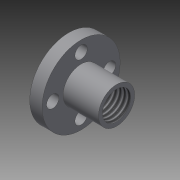
# Autodesk Inventor part: stage
Saved by Autodesk Inventor 2015 SP1 (Build 190203100, 203)
## iProperties
Created: 2016-07-08
Part Number: stage
Material: Generic
Document SubType Name: Modeling
Designer: lustinga
Density: 1 g/cm^3
Appearance: Default
Mass: 1.38148 g
Surface Area: 17.2411 cm^2
Volume: 1.38148 cm^3
Author: lustinga
Autodesk Inventor part; units mm, degrees
ref_plane "YZ Plane" through (0, 0, 0) normal (1, 0, 0) x (0, 1, 0)
ref_plane "XZ Plane" through (0, 0, 0) normal (0, 1, 0) x (-1, 0, 0)
ref_plane "XY Plane" through (0, 0, 0) normal (0, 0, 1) x (1, 0, 0)
sketch "Sketch1" plane through (0, 0, 0) normal (1, 0, 0) x (0, 1, 0)
  circle A0 centre (0, 0) radius 11
  circle A1 centre (0, 0) radius 4
  circle A2 centre (0, 0) radius 8 construction
  circle A3 centre (-8, 0) radius 1.75
  circle A4 centre (0, -8) radius 1.75
  circle A5 centre (8, 0) radius 1.75
  circle A6 centre (0, 8) radius 1.75
  dimension "d0" = 22
  dimension "d11" = 8
  dimension "d13" = 3.5
  dimension "d16" = 360
  dimension "d20" = 8
  constraints: 6 centre point, 3 coincident, 1 horizontal alignment, 11 other
  measures "d0" diameter of A0
  measures "d11" diameter of A1
  measures "d13" diameter of A3
  measures "d20" distance of point (0, 0) A5.centre
extrude "Extrusion1" add sketch "Sketch1" along normal blind 3.5
sketch "Sketch2" plane through (3.5, 0, 0) normal (1, 0, 0) x (0, 0, -1)
  circle A0 centre (0, 0) radius 5.1
  circle A1 centre (0, 0) radius 4
  dimension "d5" = 10.2
  dimension "d10" = 8
  constraints: 2 centre point, 2 coincident
  measures "d5" diameter of A0
  measures "d10" diameter of A1
extrude "Extrusion2" add sketch "Sketch2" along normal blind 10 and the other way blind 5
thread "Thread1" size "M8x1.25" class "6H" standard "ANSI Metric M Profile" full length
body "Solid1"
